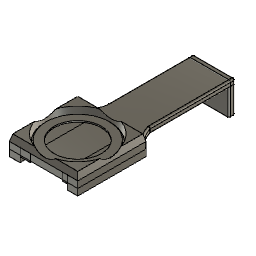
Cross Slide (Autodesk Fusion 360 design; units mm, degrees)
Autodesk Fusion 360 part; units mm, degrees
note: some values were not read from the file. Set by a fixed rule: which face or edge a step refers to.
sketch "Sketch1" plane through (0, 0, 0) normal (0, 0, 1) x (1, 0, 0)
  line L0 (0, 0) -> (82.55, 0)
  line L1 (82.55, 0) -> (82.55, 82.55)
  line L2 (69.85, 203.2) -> (19.05, 203.2)
  line L3 (0, 82.55) -> (0, 0)
  line L4 (82.55, 82.55) -> (0, 82.55)
  line L5 (19.05, 203.2) -> (19.05, 82.55)
  line L6 (69.85, 203.2) -> (69.85, 82.55)
  spline S0 degree 5 poles (0, 82.55) (0.7459, 82.6307) (2.2067, 82.8157) (4.3044, 83.1635) (6.9115, 83.7702) (9.8316, 84.7838) (12.3805, 86.0771) (14.524, 87.6758) (16.2368, 89.5989) (17.5261, 91.841) (18.4201, 94.381) (18.8428, 96.6332) (19.0054, 98.4387) (19.0464, 99.6932) (19.05, 100.3332) knots 0 0 0 0 0 0 0.1 0.2 0.3 0.4 0.5 0.6 0.7 0.8 0.9 1 1 1 1 1 1
  spline S1 degree 5 poles (82.55, 82.55) (82.19, 82.7631) (81.4794, 83.2015) (80.4419, 83.8959) (79.1163, 84.8967) (77.5617, 86.2807) (76.1181, 87.8087) (74.7935, 89.4909) (73.59, 91.3305) (72.5008, 93.3184) (71.5164, 95.4422) (70.8054, 97.2405) (70.3123, 98.6414) (70.0012, 99.5982) (69.85, 100.0822) knots 0 0 0 0 0 0 0.1 0.2 0.3 0.4 0.5 0.6 0.7 0.8 0.9 1 1 1 1 1 1
  line L7 (12.7, 82.55) -> (12.7, 0)
  line L8 (69.85, 0) -> (69.85, 82.55)
  circle A0 centre (41.275, 41.275) radius 6.35
  circle A1 centre (41.275, 41.275) radius 28.575
  circle A2 centre (41.275, 41.275) radius 38.1
  line L9 (19.05, 195.2625) -> (69.85, 195.2625)
  line L10 (25.4, 82.55) -> (25.4, 0)
  line L11 (63.5, 82.55) -> (63.5, 0)
  circle A3 centre (41.275, 41.275) radius 39.6875
  point P0 (14.8889, 88.2109)
  point P1 (75.1173, 89.1297)
  dimension "d1" = 82.55
  dimension "d3" = 82.55
  dimension "d4" = 19.05
  dimension "d5" = 12.7
  dimension "d6" = 12.7
  dimension "d7" = 12.7
  dimension "d8" = 12.7
  dimension "d9" = 41.275
  dimension "d10" = 41.275
  dimension "d11" = 57.15
  dimension "d12" = 76.2
  dimension "d13" = 7.9375
  dimension "d15" = 12.7
  dimension "d16" = 6.35
  dimension "d32" = 79.375
  constraint horizontal L0
  constraint vertical L1
  constraint horizontal L2
  constraint vertical L3
  constraint coincident L0.start L3.end
  constraint perpendicular L3 L4
  constraint coincident L4 L5.end
  constraint perpendicular L4 L5
  constraint coincident L4 L6.end
  constraint perpendicular L2 L6
  constraint coincident L5 S0.end
  constraint coincident L6 S1.end
  constraint coincident L4 L7.start
  constraint coincident L0 L7.end
  constraint perpendicular L0 L7
  constraint coincident L0 L8.start
  constraint perpendicular L4 L8
  constraint concentric A0 A1
  constraint concentric A1 A2
  constraint coincident L5 L9.start
  constraint coincident L6 L9.end
  constraint perpendicular L6 L9
  constraint coincident L4 L10.start
  constraint coincident L0 L10.end
  constraint perpendicular L0 L10
  constraint coincident L4 L11.start
  constraint coincident L0 L11.end
  constraint perpendicular L0 L11
  constraint concentric A0 A3
  measures "d1" distance of L0.start L0.end
  measures "d3" distance of L0 L4
  measures "d4" distance of L3 L5
  measures "d5" distance of L1 L6
  measures "d6" distance of L3 L7
  measures "d7" distance of L1 L8
  measures "d8" diameter of A0
  measures "d9" distance of L0 A0.centre
  measures "d10" distance of L3 A0.centre
  measures "d11" diameter of A1
  measures "d12" diameter of A2
  measures "d13" distance of L2 L9
  measures "d15" distance of L7 L10
  measures "d16" distance of L8 L11
  measures "d32" diameter of A3
extrude "Extrude1" add sketch "Sketch1" against normal blind 7.9375 contours L0 L3 L4 L7 A3 | L0 L7 L10 A3 | L4 L5 S0 | L0 L10 L11 A3 | L7 A2 A3 | L7 A2 L10 A3 | L4 L7 L10 A3 | L4 L5 L6 L9 | L0 L8 L11 A3 | A2 L10 L11 A3 | L7 A2 | L7 A1 A2 L10 | L7 A2 L10 A3 | L2 L5 L6 L9 | L0 L1 L4 L8 A3 | L8 A2 L11 A3 | A1 A2 L10 L11 | L7 A1 A2 L10 | A1 L10 | A2 L10 L11 A3 | L4 L10 L11 A3 | L8 A2 A3 | L8 A1 A2 L11 | A1 L10 L11 | A1 A2 L10 L11 | L8 A2 L11 A3 | L4 L8 L11 A3 | L4 L6 S1 | L8 A2 | A1 L11 | L8 A1 A2 L11 | A0 makes body 1
extrude "Extrude2" add sketch "Sketch1" against normal blind 9.525 separate body contours L0 L7 L10 A3 | L7 A2 L10 A3 | L4 L7 L10 A3 | L7 A1 A2 L10 | L7 A2 L10 A3 | L7 A1 A2 L10 | A1 L10 makes body 2
extrude "Extrude3" add sketch "Sketch1" against normal blind 9.525 separate body contours L0 L8 L11 A3 | L8 A2 L11 A3 | L8 A1 A2 L11 | L8 A2 L11 A3 | L4 L8 L11 A3 | A1 L11 | L8 A1 A2 L11 makes body 3
extrude "Extrude4" add sketch "Sketch1" against normal blind 15.875 separate body contours L0 L3 L4 L7 A3 | L7 A2 A3 | L7 A2 makes body 4
extrude "Extrude5" add sketch "Sketch1" against normal blind 15.875 separate body contours L0 L1 L4 L8 A3 | L8 A2 A3 | L8 A2 makes body 5
extrude "Extrude6" add sketch "Sketch1" against normal blind 39.6875 separate body contours L2 L5 L6 L9 makes body 6
extrude "Extrude7" add sketch "Sketch1" along normal blind 1.5875 separate body contours L7 A2 | L7 A1 A2 L10 | A1 A2 L10 L11 | L7 A1 A2 L10 | L8 A1 A2 L11 | A1 A2 L10 L11 | L8 A2 | L8 A1 A2 L11 makes body 7
ref_plane "WorkPlane1" through (0, 0, 7.9375) normal (0, 0, 1) x (1, 0, 0)
sketch "Sketch2" plane through (0, 0, 7.9375) normal (0, 0, 1) x (1, 0, 0)
  circle A0 centre (41.275, 41.275) radius 41.275
  point P0 (41.275, 41.275)
  dimension "d34" = 82.55
  constraint coincident P0 A0.centre
  measures "d34" diameter of A0
extrude "Extrude8" add sketch "Sketch1" along normal blind 7.9375 draft -14 separate body contours L0 L3 L4 L7 A3 | L0 L7 L10 A3 | L0 L10 L11 A3 | L7 A2 A3 | L7 A2 L10 A3 | L4 L7 L10 A3 | L0 L8 L11 A3 | A2 L10 L11 A3 | L7 A2 | L7 A1 A2 L10 | L7 A2 L10 A3 | L0 L1 L4 L8 A3 | L8 A2 L11 A3 | A1 A2 L10 L11 | L7 A1 A2 L10 | A1 L10 | A2 L10 L11 A3 | L4 L10 L11 A3 | L8 A2 A3 | L8 A1 A2 L11 | A1 L10 L11 | A1 A2 L10 L11 | L8 A2 L11 A3 | L4 L8 L11 A3 | L8 A2 | A1 L11 | L8 A1 A2 L11 | A0 makes body 8
sketch "Sketch3" plane through (0, 0, 0) normal (0, 0, 1) x (1, 0, 0)
  circle A0 centre (41.275, 41.275) radius 39.6875
  point P0 (41.275, 41.275)
  dimension "d37" = 79.375
  constraint coincident P0 A0.centre
  measures "d37" diameter of A0
loft "Loft1" cut profiles "Sketch2", "Sketch3" section 1 section 2 bodies 8
fillet "Fillet1" radius 2 4 faces at (69.85, 163.5357, -2.6458) (69.85, 200.5542, -2.6458) (70.7444, 97.4637, -2.6458) (69.85, 200.5542, -13.2292) on bodies 1 6
fillet "Fillet2" radius 2 6 edges at (69.2642, 195.8483, -39.1017) (43.45, 195.2625, -39.6875) (43.45, 203.2, -39.6875) (69.2642, 202.6142, -39.1017) (19.05, 203.2, -19.8438) (19.05, 195.2625, -19.8438) on bodies 6
fillet "Fillet3" radius 2 2 faces at (19.05, 168.9111, -2.6458) (3.4122, 83.0416, -2.6458) on bodies 1
fillet "Fillet4" radius 2 3 edges at (69.2642, 202.6142, -0.5858) (44.45, 203.2, 0) (19.6358, 202.6142, -0.5858) on bodies 1
fillet "Fillet5" radius 2 7 edges at (69.2642, 202.6142, -0.5858) (44.45, 203.2, 0) (19.6358, 202.6142, 0) (19.05, 199.2313, 0) (19.6358, 195.8483, 0) (44.45, 195.2625, 0) (69.2642, 195.8483, -0.5858) on bodies 6
